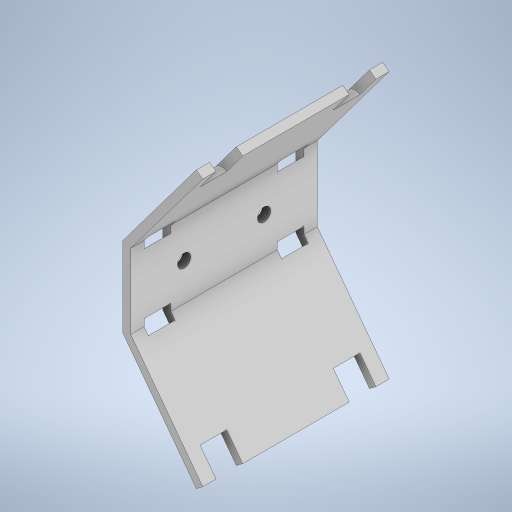
# Autodesk Inventor part: onTubeFixationTiny
Saved by Autodesk Inventor 2024 (Build 280153000, 153)
## iProperties
Created: 2023-07-05
Part Number: onTubeFixationTiny
Material: Generic
Document SubType Name: Sheet Metal
Designer: pablo
Density: 1 g/cm^3
Sheet Metal Rule: Default_mm
Appearance: Default
Author: pablo
Autodesk Inventor part; units mm, degrees
sketch "Sketch2" plane through (0, 0, 0) normal (0, 0, 1) x (1, 0, 0)
  line L0 (0, 0) -> (-30, 40)
  line L1 (-30, 40) -> (-30, 70)
  line L2 (-30, 70) -> (0, 110)
  line L3 (0, 110) -> (0, 0)
  line L4 (-2.4, 106.8) -> (0, 105)
  line L5 (-2.4, 3.2) -> (0, 5)
  dimension "d4" = 30
  dimension "d5" = 40
  dimension "d6" = 40
  dimension "d7" = 30
  dimension "d11" = 3
  dimension "d12" = 3
  constraints: 12 end point, 4 point on line, 2 perpendicular, 1 parallel, 1 vertical
  measures "d4" distance between parallel lines of L3 L1
  measures "d5" vertical distance of L2.end L1.end
  measures "d6" vertical distance of L0.start L0.end
  measures "d7" distance of L1.end L0.end
  measures "d11" distance of L4.start L4.end
  measures "d12" distance of L5.start L5.end
extrude "Extrusion2" add sketch "Sketch2" along normal mid plane 70 contours L0 L1 L2 L4 L3 L5
shell "Shell1" thickness 3 removed faces 5 at (-10, 60, -35) at (0, 71.6667, 11.6667) at (-10, 60, 35) at (-0.8, 105.6, -11.6667) at (-0.8, 4.4, 11.6667)
sketch "Sketch4" plane through (-2.4, 3.2, -35) normal (-0.8, -0.6, 0) x (0, 0, 1)
  line L0 (0, 0) -> (70, 0) projected
  line L1 (5, 0) -> (15, 0)
  line L2 (15, 0) -> (15, 10)
  line L3 (15, 10) -> (5, 10)
  line L4 (5, 10) -> (5, 0)
  line L5 (55, 0) -> (65, 0)
  line L6 (65, 0) -> (65, 10)
  line L7 (65, 10) -> (55, 10)
  line L8 (55, 10) -> (55, 0)
  line L9 (70, 46) -> (70, 0) projected
  line L10 (0, 0) -> (0, 46) projected
  point P0 (35, -4)
  point P1 (70, 54.2734)
  point P2 (0, 54.2734)
  dimension "d54" = 10
  dimension "d55" = 10
  dimension "d56" = 5
  dimension "d57" = 5
  dimension "d58" = 10
  dimension "d59" = 10
  constraints: 16 end point, 4 parallel, 2 horizontal, 2 perpendicular, 2 point on line
  measures "d54" distance between parallel lines of L4 L2
  measures "d55" distance between parallel lines of L6 L8
  measures "d56" distance between parallel lines of L9 L6
  measures "d57" distance between parallel lines of L10 L4
  measures "d58" distance between parallel lines of L0 L3
  measures "d59" distance between parallel lines of L0 L7
extrude "Extrusion3" cut sketch "Sketch4" against normal through all
sketch "Sketch5" plane through (-2.4, 106.8, -35) normal (-0.8, 0.6, 0) x (0, 0, 1)
  line L0 (0, 0) -> (70, 0) projected
  line L1 (65, 0) -> (55, 0)
  line L2 (55, 0) -> (55, -10)
  line L3 (55, -10) -> (65, -10)
  line L4 (65, -10) -> (65, 0)
  line L5 (5, 0) -> (15, 0)
  line L6 (15, 0) -> (15, -10)
  line L7 (15, -10) -> (5, -10)
  line L8 (5, -10) -> (5, 0)
  line L9 (0, -46) -> (0, 0) projected
  line L10 (70, 0) -> (70, -46) projected
  point P0 (35, -84)
  point P1 (0, -54.2734)
  point P2 (70, -54.2734)
  point P3 (15, 0)
  point P4 (55, 0)
  dimension "d62" = 5
  dimension "d63" = 5
  dimension "d64" = 10
  dimension "d65" = 10
  dimension "d66" = 10
  constraints: 16 end point, 4 parallel, 3 point on line, 2 horizontal, 2 perpendicular
  measures "d62" distance between parallel lines of L9 L8
  measures "d63" distance between parallel lines of L10 L4
  measures "d64" distance between parallel lines of L2 L4
  measures "d65" distance between parallel lines of L8 L6
  measures "d66" distance between parallel lines of L0 L3
extrude "Extrusion4" cut sketch "Sketch5" against normal through all
fillet "Fillet3" radius 3 4 edges at (-8.4, 98.8, -25) (-8.4, 98.8, 25) (-8.4, 11.2, -25) (-8.4, 11.2, 25)
ref_plane "Work Plane1" through (-30, 70, -35) normal (0.3162278, 0.9486833, 0) x (0, 0, -1)
ref_plane "Work Plane2" through (-30, 40, -35) normal (0.3162278, -0.9486833, 0) x (0, 0, 1)
sketch "Sketch8" plane through (-30, 70, -35) normal (0.3162278, 0.9486833, 0) x (0, 0, -1)
  line L0 (0, 0) -> (-70, 0) projected
  line L1 (-65, 0) -> (-55, 0)
  line L2 (-55, 0) -> (-55, -4)
  line L3 (-55, -4) -> (-65, -4)
  line L4 (-65, -4) -> (-65, 0)
  line L5 (-70, -12.0167) -> (-70, -3.1623) projected
  line L6 (-15, 0) -> (-5, 0)
  line L7 (-5, 0) -> (-5, -4)
  line L8 (-5, -4) -> (-15, -4)
  line L9 (-15, -4) -> (-15, 0)
  line L10 (0, -9.4868) -> (0, 0) projected
  point P0 (-35, -50.5964)
  dimension "d87" = 10
  dimension "d88" = 5
  dimension "d89" = 4
  dimension "d90" = 5
  dimension "d91" = 10
  dimension "d92" = 4
  constraints: 16 end point, 4 parallel, 2 horizontal, 2 perpendicular, 2 point on line
  measures "d87" distance between parallel lines of L2 L4
  measures "d88" distance between parallel lines of L5 L4
  measures "d89" distance between parallel lines of L3 L0
  measures "d90" distance between parallel lines of L10 L7
  measures "d91" distance between parallel lines of L7 L9
  measures "d92" distance between parallel lines of L0 L8
extrude "Extrusion5" cut sketch "Sketch8" along normal through all both and the other way through all
ref_plane "Work Plane3" through (-41.25, 55, -20) normal (0, 1, 0) x (0, 0, -1)
mirror "Mirror1" about plane through (-41.25, 55, -20) normal (0, 1, 0) of "Extrusion5"
sketch "Sketch9" plane through (-30, 40, 35) normal (-1, 0, 0) x (0, 0, 1)
  line L0 (-70, 0) -> (-70, 30) projected
  line L1 (0, 30) -> (0, 0) projected
  line L2 (-70, 0) -> (0, 30)
  line L3 (-70, 30) -> (-65, 30) projected
  line L4 (0, 0) -> (-70, 30)
  line L5 (-35, 15) -> (0, 15)
  line L6 (-35, 15) -> (-70, 15)
  line L7 (-35, 15) -> (-35, 30)
  line L8 (-55, 30) -> (-15, 30) projected
  line L9 (-35, 15) -> (-35, 0)
  line L10 (-15, 0) -> (-55, 0) projected
  line L11 (-50, 15) -> (-35, 30)
  line L12 (-20, 15) -> (-35, 0)
  line L13 (-35, 0) -> (-50, 15)
  line L14 (-20, 15) -> (-35, 30)
  point P0 (-35, -40)
  dimension "d95" = 30
  dimension "d96" = 30
  constraints: 20 end point, 5 midpoint, 4 point on line, 3 perpendicular
  measures "d95" distance of L11.end L12.end
  measures "d96" distance of L12.start L11.start
hole "Hole2" at (-30, 55, 15) at (-30, 55, -15) direction (1, 0, 0) diameter 5 depth 5
thread "Thread8" size "M5x0.8" class "6H" standard "ANSI Metric M Profile" full length
thread "Thread9" size "M5x0.8" class "6H" standard "ANSI Metric M Profile" full length
equation "\"d102\" = Thickness"
equation "\"BendRadius\" = Thickness"
equation "\"BendReliefWidth\" = Thickness"
equation "\"BendReliefDepth\" = 0.5 * Thickness"
equation "\"TransitionRadius\" = BendRadius"
equation "\"JacobiRadiusSize\" = BendRadius"
equation "\"GapSize\" = Thickness"
equation "\"d13\" = Thickness"
equation "\"Thickness\" = 5"
body "Solid2"
